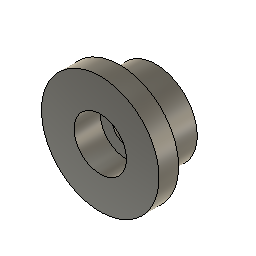
rotoforgewireguide v13 (Autodesk Fusion 360 archive; units mm, degrees)
design "sawbladeclamparborend"
Autodesk Fusion 360 part; units mm, degrees
sketch "Sketch1" plane through (0, 0, 0) normal (0, 1, 0) x (1, 0, 0)
  circle A0 centre (0, 0) radius 6.35
  dimension "d1" = 12.7
  constraint coincident A0.centre origin
  measures "d1" diameter of A0
extrude "Extrude1" add sketch "Sketch1" along normal blind 5.5
sketch "Sketch2" plane through (0, 0, 0) normal (0, -1, 0) x (1, 0, 0)
  circle A0 centre (0, 0) radius 6.35
  circle A1 centre (0, 0) radius 9
  dimension "d4" = 18
  constraint coincident A0.centre A1.centre
  measures "d4" diameter of A1
extrude "Extrude2" add sketch "Sketch2" along normal blind 3 contours A0 | A1
sketch "Sketch3" plane through (0, -3, 0) normal (0, -1, 0) x (1, 0, 0)
  circle A0 centre (0, 0) radius 9
  circle A1 centre (0, 0) radius 2
  dimension "d7" = 4
  constraint coincident A0.centre A1.centre
  measures "d7" diameter of A1
hole "Hole1" at (0, -3, 0) direction (0, 1, 0) diameter 4.3 end through all counterbore diameter 8 counterbore depth 4
equation "d1 = 0'- 1/2\""

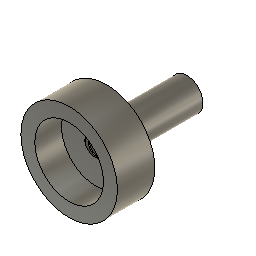
design "RotoforgeArbor"
Autodesk Fusion 360 part; units mm, degrees
sketch "Sketch1" plane through (0, 0, 0) normal (0, 1, 0) x (1, 0, 0)
  circle A0 centre (0, 0) radius 3
  dimension "d1" = 6
  constraint coincident A0.centre origin
  measures "d1" diameter of A0
extrude "Extrude1" add sketch "Sketch1" along normal blind 13
sketch "Sketch2" plane through (0, 0, 0) normal (0, -1, 0) x (1, 0, 0)
  circle A0 centre (0, 0) radius 3
  circle A1 centre (0, 0) radius 9
  dimension "d4" = 18
  constraint concentric A0 A1
  measures "d4" diameter of A1
extrude "Extrude2" add sketch "Sketch2" along normal blind 7 contours A0 | A1
sketch "Sketch3" plane through (0, -7, 0) normal (0, -1, 0) x (1, 0, 0)
  circle A0 centre (0, 0) radius 9
  circle A1 centre (0, 0) radius 6.4
  dimension "d7" = 12.8
  constraint concentric A0 A1
  measures "d7" diameter of A1
extrude "Extrude3" cut sketch "Sketch3" against normal blind 5 contours A1
sketch "Sketch4" plane through (0, -2, 0) normal (0, -1, 0) x (1, 0, 0)
  circle A0 centre (0, 0) radius 6.4
  circle A1 centre (0, 0) radius 2
  dimension "d10" = 4
  constraint coincident A0.centre A1.centre
  measures "d10" diameter of A1
hole "Hole1" at (0, -2, 0) direction (0, 1, 0) diameter 3.332 depth 5 tip angle 118
thread "Thread1" "ISO Metric profile 4.0 M4x0.7 M4x0.7 6H" major diameter 4.1095 minor diameter 3.332 pitch 0.7 angle 60 modelled right hand crest width 0.193 on face at (0.083, -0.3333, -1.6639) crest through (0, -1.825, -1.666)
chamfer "Chamfer1" distance 3 angle 45 1 edges at (-2.797, 0, 1.0848)
extrude "Extrude4" add 1 faces at (0.3505, 13, 0.866) along direction (0, 1, 0) blind 2

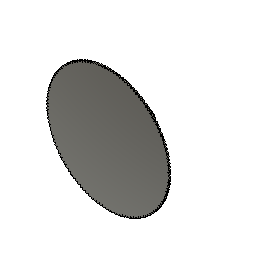
design "RotoforgewheelV9"
Autodesk Fusion 360 part; units mm, degrees
sketch "Sketch1" plane through (0, 0, 0) normal (0, 1, 0) x (1, 0, 0)
  circle A0 centre (0, 0) radius 3.2
  dimension "d1" = 6.4
  constraint coincident A0.centre origin
  measures "d1" diameter of A0
extrude "Extrude1" add sketch "Sketch1" along normal blind 13.77 makes body 1
sketch "Sketch2" plane through (0, 0, 0) normal (0, -1, 0) x (1, 0, 0)
  circle A0 centre (0, 0) radius 3.2
  circle A1 centre (0, 0) radius 3.2
  constraint coincident A0.centre A1.centre
  constraint equal A0 A1
extrude "Extrude2" add sketch "Sketch2" along normal blind 2.5 separate body makes body 2
sketch "Sketch3" plane through (0, -2.5, 0) normal (0, -1, 0) x (1, 0, 0)
  circle A0 centre (0, 0) radius 3.2
  circle A1 centre (0, 0) radius 25.85
  dimension "d7" = 51.7
  constraint coincident A0.centre A1.centre
  measures "d7" diameter of A1
extrude "Extrude3" add sketch "Sketch3" along normal blind 0.65 contours A0 | A1 bodies 2
sketch "Sketch4" plane through (0, -3.15, 0) normal (0, -1, 0) x (1, 0, 0)
  circle A0 centre (0, 0) radius 25.85
  line L0 (1.75, 0) -> (22.5, 0)
  line L1 (0, 1.75) -> (0, 22.5)
  line L2 (-0.35, 25.8476) -> (0, 25.3)
  line L3 (0, 25.3) -> (0.35, 25.8476)
  dimension "d10" = 0.7
  dimension "d11" = 2.8
  constraint coincident A0 L2.start
  constraint coincident A0 L3.end
  constraint coincident L1 L2.end
  constraint symmetric L1 L2 L3
  measures "d10" horizontal distance of L2.start L3.end
  measures "d11" distance of L1.end L2.end
extrude "Extrude4" cut sketch "Sketch4" against normal up to surface (0.65 mm away) contours A0 L2 L3 picked at (0, 25.6665) bodies 2
pattern_circular "C-Pattern1" count 130 over 360 about axis through (0, 1.75, 0) along (0, 1, 0) of "Extrude4"
combine "Combine1" operation add target body 1 tool bodies 2
fillet "Fillet1" radius 1.5 1 edges at (-2.9834, -2.5, -1.1572) on bodies 1
